Autodesk Inventor part; units mm, degrees
(part 8 of 15)
  arc A3405 (-52.178, -58.6781) -> (-52.178, -58.6019) centre (-52.178, -58.64) ccw
  arc A3406 (-55.022, -58.6019) -> (-55.022, -58.6781) centre (-55.022, -58.64) ccw
  line L1559 (-52.178, -58.64) -> (-52.178, -59.96)
  arc A3407 (-52.2161, -59.96) -> (-52.1399, -59.96) centre (-52.178, -59.96) ccw
  arc A3408 (-52.1399, -58.64) -> (-52.2161, -58.64) centre (-52.178, -58.64) ccw
  line L1560 (-52.178, -59.96) -> (-55.022, -59.96)
  arc A3409 (-55.022, -59.9219) -> (-55.022, -59.9981) centre (-55.022, -59.96) ccw
  arc A3410 (-52.178, -59.9981) -> (-52.178, -59.9219) centre (-52.178, -59.96) ccw
  line L1561 (-18.1, 57.4) -> (-18.1, 55)
  arc A3411 (-18.1317, 55) -> (-18.0682, 55) centre (-18.1, 55) ccw
  arc A3412 (-18.0682, 57.4) -> (-18.1317, 57.4) centre (-18.1, 57.4) ccw
  line L1562 (-18.1, 55) -> (-19.1, 55)
  arc A3413 (-19.1, 55.0318) -> (-19.1, 54.9683) centre (-19.1, 55) ccw
  arc A3414 (-18.1, 54.9683) -> (-18.1, 55.0318) centre (-18.1, 55) ccw
  line L1563 (-19.1, 55) -> (-19.1, 57.4)
  arc A3415 (-19.0682, 57.4) -> (-19.1317, 57.4) centre (-19.1, 57.4) ccw
  arc A3416 (-19.1317, 55) -> (-19.0682, 55) centre (-19.1, 55) ccw
  line L1564 (-19.1, 57.4) -> (-18.1, 57.4)
  arc A3417 (-18.1, 57.3683) -> (-18.1, 57.4317) centre (-18.1, 57.4) ccw
  arc A3418 (-19.1, 57.4317) -> (-19.1, 57.3683) centre (-19.1, 57.4) ccw
  line L1565 (-4.8, -82.3) -> (-4.8, -85.1)
  arc A3419 (-4.8318, -85.1) -> (-4.7682, -85.1) centre (-4.8, -85.1) ccw
  arc A3420 (-4.7682, -82.3) -> (-4.8318, -82.3) centre (-4.8, -82.3) ccw
  line L1566 (-6.6, -85.1) -> (-6.6, -82.3)
  arc A3421 (-6.5682, -82.3) -> (-6.6317, -82.3) centre (-6.6, -82.3) ccw
  arc A3422 (-6.6317, -85.1) -> (-6.5682, -85.1) centre (-6.6, -85.1) ccw
  line L1567 (-16.5, -87.6) -> (-16.5, -90.4)
  arc A3423 (-16.5318, -90.4) -> (-16.4683, -90.4) centre (-16.5001, -90.4) ccw
  arc A3424 (-16.4683, -87.6) -> (-16.5318, -87.6) centre (-16.5001, -87.6) ccw
  line L1568 (-18.3, -90.4) -> (-18.3, -87.6)
  arc A3425 (-18.2682, -87.6) -> (-18.3318, -87.6) centre (-18.3, -87.6) ccw
  arc A3426 (-18.3318, -90.4) -> (-18.2682, -90.4) centre (-18.3, -90.4) ccw
  line L1569 (-13.675, -20.475) -> (-13.675, -23.125)
  arc A3427 (-13.7004, -23.125) -> (-13.6496, -23.125) centre (-13.675, -23.125) ccw
  arc A3428 (-13.6496, -20.475) -> (-13.7004, -20.475) centre (-13.675, -20.475) ccw
  line L1570 (-12.125, -20.475) -> (-12.125, -23.125)
  arc A3429 (-12.1504, -23.125) -> (-12.0996, -23.125) centre (-12.125, -23.125) ccw
  arc A3430 (-12.0996, -20.475) -> (-12.1504, -20.475) centre (-12.125, -20.475) ccw
  line L1571 (-12.9, -21.3) -> (-12.4, -22.3)
  arc A3431 (-12.4454, -22.3227) -> (-12.3546, -22.2773) centre (-12.4, -22.3) ccw
  arc A3432 (-12.8546, -21.2773) -> (-12.9454, -21.3227) centre (-12.9, -21.3) ccw
  line L1572 (-12.4, -22.3) -> (-13.4, -22.3)
  arc A3433 (-13.4, -22.2492) -> (-13.4, -22.3508) centre (-13.4, -22.3) ccw
  arc A3434 (-12.4, -22.3508) -> (-12.4, -22.2492) centre (-12.4, -22.3) ccw
  line L1573 (-13.4, -22.3) -> (-12.9, -21.3)
  arc A3435 (-12.8546, -21.3227) -> (-12.9454, -21.2773) centre (-12.9, -21.3) ccw
  arc A3436 (-13.4454, -22.2773) -> (-13.3546, -22.3227) centre (-13.4, -22.3) ccw
  line L1574 (-12.4, -21.3) -> (-12.9, -21.3)
  arc A3437 (-12.9, -21.2492) -> (-12.9, -21.3508) centre (-12.9, -21.3) ccw
  arc A3438 (-12.4, -21.3508) -> (-12.4, -21.2492) centre (-12.4, -21.3) ccw
  line L1575 (-12.9, -21.3) -> (-13.4, -21.3)
  arc A3439 (-13.4, -21.2492) -> (-13.4, -21.3508) centre (-13.4, -21.3) ccw
  arc A3440 (-12.9, -21.3508) -> (-12.9, -21.2492) centre (-12.9, -21.3) ccw
  line L1576 (-15.6, 42.2) -> (-17.4, 42.2)
  arc A3441 (-17.4, 42.2317) -> (-17.4, 42.1683) centre (-17.4, 42.2) ccw
  arc A3442 (-15.6, 42.1683) -> (-15.6, 42.2317) centre (-15.6, 42.2) ccw
  line L1577 (-17.4, 43.6) -> (-15.6, 43.6)
  arc A3443 (-15.6, 43.5683) -> (-15.6, 43.6318) centre (-15.6, 43.6) ccw
  arc A3444 (-17.4, 43.6318) -> (-17.4, 43.5683) centre (-17.4, 43.6) ccw
  line L1578 (-17.4, 42.2) -> (-17.4, 43.6)
  arc A3445 (-17.3682, 43.6) -> (-17.4317, 43.6) centre (-17.4, 43.6) ccw
  arc A3446 (-17.4317, 42.2) -> (-17.3682, 42.2) centre (-17.4, 42.2) ccw
  line L1579 (-16.7, 42.23) -> (-16.7, 43.5)
  arc A3447 (-16.6682, 43.5) -> (-16.7317, 43.5) centre (-16.7, 43.5) ccw
  arc A3448 (-16.7317, 42.23) -> (-16.6682, 42.23) centre (-16.7, 42.23) ccw
  line L1580 (-15.6, 43.6) -> (-15.6, 42.2)
  arc A3449 (-15.6317, 42.2) -> (-15.5682, 42.2) centre (-15.6, 42.2) ccw
  arc A3450 (-15.5682, 43.6) -> (-15.6317, 43.6) centre (-15.6, 43.6) ccw
  line L1581 (16.64, -104.878) -> (17.96, -104.878)
  arc A3451 (17.96, -104.9161) -> (17.96, -104.8399) centre (17.96, -104.878) ccw
  arc A3452 (16.64, -104.8399) -> (16.64, -104.9161) centre (16.64, -104.878) ccw
  line L1582 (17.96, -104.878) -> (17.96, -107.722)
  arc A3453 (17.9219, -107.722) -> (17.9981, -107.722) centre (17.96, -107.722) ccw
  arc A3454 (17.9981, -104.878) -> (17.9219, -104.878) centre (17.96, -104.878) ccw
  line L1583 (17.96, -107.722) -> (16.64, -107.722)
  arc A3455 (16.64, -107.6839) -> (16.64, -107.7601) centre (16.64, -107.722) ccw
  arc A3456 (17.96, -107.7601) -> (17.96, -107.6839) centre (17.96, -107.722) ccw
  line L1584 (16.64, -107.722) -> (16.64, -104.878)
  arc A3457 (16.6781, -104.878) -> (16.6019, -104.878) centre (16.64, -104.878) ccw
  arc A3458 (16.6019, -107.722) -> (16.6781, -107.722) centre (16.64, -107.722) ccw
  line L1585 (66.55, 47.1) -> (69.05, 47.1)
  arc A3459 (69.05, 47.075) -> (69.05, 47.125) centre (69.05, 47.1) ccw
  arc A3460 (66.55, 47.125) -> (66.55, 47.075) centre (66.55, 47.1) ccw
  line L1586 (69.05, 46.1) -> (66.55, 46.1)
  arc A3461 (66.55, 46.125) -> (66.55, 46.075) centre (66.55, 46.1) ccw
  arc A3462 (69.05, 46.075) -> (69.05, 46.125) centre (69.05, 46.1) ccw
  line L1587 (69.05, 47.1) -> (69.05, 46.1)
  arc A3463 (69.025, 46.1) -> (69.075, 46.1) centre (69.05, 46.1) ccw
  arc A3464 (69.075, 47.1) -> (69.025, 47.1) centre (69.05, 47.1) ccw
  line L1588 (66.55, 46.1) -> (66.55, 47.1)
  arc A3465 (66.575, 47.1) -> (66.525, 47.1) centre (66.55, 47.1) ccw
  arc A3466 (66.525, 46.1) -> (66.575, 46.1) centre (66.55, 46.1) ccw
  arc A3467 (68.7, 46.75) -> (68.7, 46.85) centre (68.7, 46.8) ccw
  arc A3468 (68.7, 46.85) -> (68.7, 46.75) centre (68.7, 46.8) ccw
  line L1589 (64.6, 38.15) -> (64.6, 40.65)
  arc A3469 (64.625, 40.65) -> (64.575, 40.65) centre (64.6, 40.65) ccw
  arc A3470 (64.575, 38.15) -> (64.625, 38.15) centre (64.6, 38.15) ccw
  line L1590 (65.6, 40.65) -> (65.6, 38.15)
  arc A3471 (65.575, 38.15) -> (65.625, 38.15) centre (65.6, 38.15) ccw
  arc A3472 (65.625, 40.65) -> (65.575, 40.65) centre (65.6, 40.65) ccw
  line L1591 (64.6, 40.65) -> (65.6, 40.65)
  arc A3473 (65.6, 40.625) -> (65.6, 40.675) centre (65.6, 40.65) ccw
  arc A3474 (64.6, 40.675) -> (64.6, 40.625) centre (64.6, 40.65) ccw
  line L1592 (65.6, 38.15) -> (64.6, 38.15)
  arc A3475 (64.6, 38.175) -> (64.6, 38.125) centre (64.6, 38.15) ccw
  arc A3476 (65.6, 38.125) -> (65.6, 38.175) centre (65.6, 38.15) ccw
  arc A3477 (64.9, 40.25) -> (64.9, 40.35) centre (64.9, 40.3) ccw
  arc A3478 (64.9, 40.35) -> (64.9, 40.25) centre (64.9, 40.3) ccw
  line L1593 (-18.111, 52.3542) -> (-18.111, 50.0458)
  arc A3479 (-18.1427, 50.0458) -> (-18.0792, 50.0458) centre (-18.111, 50.0458) ccw
  arc A3480 (-18.0792, 52.3542) -> (-18.1427, 52.3542) centre (-18.111, 52.3542) ccw
  line L1594 (-18.111, 50.0458) -> (-19.089, 50.0458)
  arc A3481 (-19.089, 50.0775) -> (-19.089, 50.0141) centre (-19.089, 50.0458) ccw
  arc A3482 (-18.111, 50.0141) -> (-18.111, 50.0775) centre (-18.111, 50.0458) ccw
  line L1595 (-19.089, 50.0458) -> (-19.089, 52.3542)
  arc A3483 (-19.0572, 52.3542) -> (-19.1208, 52.3542) centre (-19.089, 52.3542) ccw
  arc A3484 (-19.1208, 50.0458) -> (-19.0572, 50.0458) centre (-19.089, 50.0458) ccw
  line L1596 (-19.089, 52.3542) -> (-18.111, 52.3542)
  arc A3485 (-18.111, 52.3225) -> (-18.111, 52.386) centre (-18.111, 52.3542) ccw
  arc A3486 (-19.089, 52.386) -> (-19.089, 52.3225) centre (-19.089, 52.3542) ccw
  line L1597 (-18.111, 54.6542) -> (-18.111, 52.3458)
  arc A3487 (-18.1427, 52.3458) -> (-18.0792, 52.3458) centre (-18.111, 52.3458) ccw
  arc A3488 (-18.0792, 54.6542) -> (-18.1427, 54.6542) centre (-18.111, 54.6542) ccw
  line L1598 (-18.111, 52.3458) -> (-19.089, 52.3458)
  arc A3489 (-19.089, 52.3776) -> (-19.089, 52.3141) centre (-19.089, 52.3458) ccw
  arc A3490 (-18.111, 52.3141) -> (-18.111, 52.3776) centre (-18.111, 52.3458) ccw
  line L1599 (-19.089, 52.3458) -> (-19.089, 54.6542)
  arc A3491 (-19.0572, 54.6542) -> (-19.1208, 54.6542) centre (-19.089, 54.6542) ccw
  arc A3492 (-19.1208, 52.3458) -> (-19.0572, 52.3458) centre (-19.089, 52.3458) ccw
  line L1600 (-19.089, 54.6542) -> (-18.111, 54.6542)
  arc A3493 (-18.111, 54.6225) -> (-18.111, 54.6859) centre (-18.111, 54.6542) ccw
  arc A3494 (-19.089, 54.6859) -> (-19.089, 54.6225) centre (-19.089, 54.6542) ccw
  line L1601 (-17.111, 56.0542) -> (-17.111, 53.7458)
  arc A3495 (-17.1427, 53.7458) -> (-17.0792, 53.7458) centre (-17.111, 53.7458) ccw
  arc A3496 (-17.0792, 56.0542) -> (-17.1427, 56.0542) centre (-17.111, 56.0542) ccw
  line L1602 (-17.111, 53.7458) -> (-18.089, 53.7458)
  arc A3497 (-18.089, 53.7775) -> (-18.089, 53.7141) centre (-18.089, 53.7458) ccw
  arc A3498 (-17.111, 53.7141) -> (-17.111, 53.7775) centre (-17.111, 53.7458) ccw
  line L1603 (-18.089, 53.7458) -> (-18.089, 56.0542)
  arc A3499 (-18.0572, 56.0542) -> (-18.1208, 56.0542) centre (-18.089, 56.0542) ccw
  arc A3500 (-18.1208, 53.7458) -> (-18.0572, 53.7458) centre (-18.089, 53.7458) ccw
  line L1604 (-18.089, 56.0542) -> (-17.111, 56.0542)
  arc A3501 (-17.111, 56.0225) -> (-17.111, 56.0859) centre (-17.111, 56.0542) ccw
  arc A3502 (-18.089, 56.0859) -> (-18.089, 56.0225) centre (-18.089, 56.0542) ccw
  line L1605 (-9.008, 3.184) -> (-9.008, 5.216)
  arc A3503 (-8.9572, 5.216) -> (-9.0588, 5.216) centre (-9.008, 5.216) ccw
  arc A3504 (-9.0588, 3.184) -> (-8.9572, 3.184) centre (-9.008, 3.184) ccw
  line L1606 (-9.008, 5.216) -> (-7.992, 5.216)
  arc A3505 (-7.992, 5.1652) -> (-7.992, 5.2668) centre (-7.992, 5.216) ccw
  arc A3506 (-9.008, 5.2668) -> (-9.008, 5.1652) centre (-9.008, 5.216) ccw
  line L1607 (-7.992, 5.216) -> (-7.992, 3.184)
  arc A3507 (-8.0428, 3.184) -> (-7.9412, 3.184) centre (-7.992, 3.184) ccw
  arc A3508 (-7.9412, 5.216) -> (-8.0428, 5.216) centre (-7.992, 5.216) ccw
  line L1608 (-7.992, 3.184) -> (-9.008, 3.184)
  arc A3509 (-9.008, 3.2348) -> (-9.008, 3.1332) centre (-9.008, 3.184) ccw
  arc A3510 (-7.992, 3.1332) -> (-7.992, 3.2348) centre (-7.992, 3.184) ccw
  line L1609 (-3.992, -3.784) -> (-3.992, -5.816)
  arc A3511 (-4.0428, -5.816) -> (-3.9412, -5.816) centre (-3.992, -5.816) ccw
  arc A3512 (-3.9412, -3.784) -> (-4.0428, -3.784) centre (-3.992, -3.784) ccw
  line L1610 (-3.992, -5.816) -> (-5.008, -5.816)
  arc A3513 (-5.008, -5.7652) -> (-5.008, -5.8668) centre (-5.008, -5.816) ccw
  arc A3514 (-3.992, -5.8668) -> (-3.992, -5.7652) centre (-3.992, -5.816) ccw
  line L1611 (-5.008, -5.816) -> (-5.008, -3.784)
  arc A3515 (-4.9572, -3.784) -> (-5.0588, -3.784) centre (-5.008, -3.784) ccw
  arc A3516 (-5.0588, -5.816) -> (-4.9572, -5.816) centre (-5.008, -5.816) ccw
  line L1612 (-5.008, -3.784) -> (-3.992, -3.784)
  arc A3517 (-3.992, -3.8348) -> (-3.992, -3.7332) centre (-3.992, -3.784) ccw
  arc A3518 (-5.008, -3.7332) -> (-5.008, -3.8348) centre (-5.008, -3.784) ccw
  line L1613 (-0.984, -4.808) -> (-3.016, -4.808)
  arc A3519 (-3.016, -4.7572) -> (-3.016, -4.8588) centre (-3.016, -4.808) ccw
  arc A3520 (-0.984, -4.8588) -> (-0.984, -4.7572) centre (-0.984, -4.808) ccw
  line L1614 (-3.016, -4.808) -> (-3.016, -3.792)
  arc A3521 (-2.9652, -3.792) -> (-3.0668, -3.792) centre (-3.016, -3.792) ccw
  arc A3522 (-3.0668, -4.808) -> (-2.9652, -4.808) centre (-3.016, -4.808) ccw
  line L1615 (-3.016, -3.792) -> (-0.984, -3.792)
  arc A3523 (-0.984, -3.8428) -> (-0.984, -3.7412) centre (-0.984, -3.792) ccw
  arc A3524 (-3.016, -3.7412) -> (-3.016, -3.8428) centre (-3.016, -3.792) ccw
  line L1616 (-0.984, -3.792) -> (-0.984, -4.808)
  arc A3525 (-1.0348, -4.808) -> (-0.9332, -4.808) centre (-0.984, -4.808) ccw
  arc A3526 (-0.9332, -3.792) -> (-1.0348, -3.792) centre (-0.984, -3.792) ccw
  line L1617 (-5.984, 5.192) -> (-8.016, 5.192)
  arc A3527 (-8.016, 5.2428) -> (-8.016, 5.1412) centre (-8.016, 5.192) ccw
  arc A3528 (-5.984, 5.1412) -> (-5.984, 5.2428) centre (-5.984, 5.192) ccw
  line L1618 (-8.016, 5.192) -> (-8.016, 6.208)
  arc A3529 (-7.9652, 6.208) -> (-8.0668, 6.208) centre (-8.016, 6.208) ccw
  arc A3530 (-8.0668, 5.192) -> (-7.9652, 5.192) centre (-8.016, 5.192) ccw
  line L1619 (-8.016, 6.208) -> (-5.984, 6.208)
  arc A3531 (-5.984, 6.1572) -> (-5.984, 6.2588) centre (-5.984, 6.208) ccw
  arc A3532 (-8.016, 6.2588) -> (-8.016, 6.1572) centre (-8.016, 6.208) ccw
  line L1620 (-5.984, 6.208) -> (-5.984, 5.192)
  arc A3533 (-6.0348, 5.192) -> (-5.9332, 5.192) centre (-5.984, 5.192) ccw
  arc A3534 (-5.9332, 6.208) -> (-6.0348, 6.208) centre (-5.984, 6.208) ccw
  line L1621 (-15.15, -102.15) -> (-15.15, -97.65)
  arc A3535 (-15.1182, -97.65) -> (-15.1817, -97.65) centre (-15.15, -97.65) ccw
  arc A3536 (-15.1817, -102.15) -> (-15.1182, -102.15) centre (-15.15, -102.15) ccw
  line L1622 (-15.15, -97.65) -> (-11.65, -97.65)
  arc A3537 (-11.65, -97.6817) -> (-11.65, -97.6182) centre (-11.65, -97.65) ccw
  arc A3538 (-15.15, -97.6182) -> (-15.15, -97.6817) centre (-15.15, -97.65) ccw
  line L1623 (-11.65, -102.15) -> (-15.15, -102.15)
  arc A3539 (-15.15, -102.1182) -> (-15.15, -102.1817) centre (-15.15, -102.15) ccw
  arc A3540 (-11.65, -102.1817) -> (-11.65, -102.1182) centre (-11.65, -102.15) ccw
  line L1624 (-11.65, -97.65) -> (-11.65, -102.15)
  arc A3541 (-11.6817, -102.15) -> (-11.6182, -102.15) centre (-11.65, -102.15) ccw
  arc A3542 (-11.6182, -97.65) -> (-11.6817, -97.65) centre (-11.65, -97.65) ccw
  arc A3543 (-14.7, -98.1) -> (-14.7, -97.9) centre (-14.7, -98) ccw
  arc A3544 (-14.7, -97.9) -> (-14.7, -98.1) centre (-14.7, -98) ccw
  line L1625 (19.6, -115) -> (16.6, -115)
  arc A3545 (16.6, -114.9682) -> (16.6, -115.0317) centre (16.6, -115) ccw
  arc A3546 (19.6, -115.0317) -> (19.6, -114.9682) centre (19.6, -115) ccw
  line L1626 (16.6, -112) -> (19.6, -112)
  arc A3547 (19.6, -112.0317) -> (19.6, -111.9682) centre (19.6, -112) ccw
  arc A3548 (16.6, -111.9682) -> (16.6, -112.0317) centre (16.6, -112) ccw
  line L1627 (19.6, -112) -> (19.6, -115)
  arc A3549 (19.5683, -115) -> (19.6318, -115) centre (19.6, -115) ccw
  arc A3550 (19.6318, -112) -> (19.5683, -112) centre (19.6, -112) ccw
  line L1628 (16.6, -115) -> (16.6, -112)
  arc A3551 (16.6318, -112) -> (16.5683, -112) centre (16.6, -112) ccw
  arc A3552 (16.5683, -115) -> (16.6318, -115) centre (16.6, -115) ccw
  arc A3553 (19.2, -112.5) -> (19.2, -112.3) centre (19.2, -112.4) ccw
  arc A3554 (19.2, -112.3) -> (19.2, -112.5) centre (19.2, -112.4) ccw
  line L1629 (-22.2, -23.7) -> (-22.2, -25.7)
  arc A3555 (-22.2318, -25.7) -> (-22.1682, -25.7) centre (-22.2, -25.7) ccw
  arc A3556 (-22.1682, -23.7) -> (-22.2318, -23.7) centre (-22.2, -23.7) ccw
  line L1630 (-24.2, -25.7) -> (-24.2, -23.7)
  arc A3557 (-24.1682, -23.7) -> (-24.2318, -23.7) centre (-24.2, -23.7) ccw
  arc A3558 (-24.2318, -25.7) -> (-24.1682, -25.7) centre (-24.2, -25.7) ccw
  arc A3559 (-21.9, -23.4) -> (-21.9, -23.2) centre (-21.9, -23.3) ccw
  arc A3560 (-21.9, -23.2) -> (-21.9, -23.4) centre (-21.9, -23.3) ccw
  line L1631 (-22.0888, 36.6332) -> (-22.0888, 38.7668)
  arc A3561 (-22.0507, 38.7668) -> (-22.1269, 38.7668) centre (-22.0888, 38.7668) ccw
  arc A3562 (-22.1269, 36.6332) -> (-22.0507, 36.6332) centre (-22.0888, 36.6332) ccw
  line L1632 (-22.0888, 38.7668) -> (-22.4952, 38.7668)
  arc A3563 (-22.4952, 38.8049) -> (-22.4952, 38.7287) centre (-22.4952, 38.7668) ccw
  arc A3564 (-22.0888, 38.7287) -> (-22.0888, 38.8049) centre (-22.0888, 38.7668) ccw
  line L1633 (-22.4952, 38.7668) -> (-22.5714, 38.7668)
  arc A3565 (-22.5714, 38.8049) -> (-22.5714, 38.7287) centre (-22.5714, 38.7668) ccw
  arc A3566 (-22.4952, 38.7287) -> (-22.4952, 38.8049) centre (-22.4952, 38.7668) ccw
  line L1634 (-22.5714, 38.7668) -> (-23.0286, 38.7668)
  arc A3567 (-23.0286, 38.8049) -> (-23.0286, 38.7287) centre (-23.0286, 38.7668) ccw
  arc A3568 (-22.5714, 38.7287) -> (-22.5714, 38.8049) centre (-22.5714, 38.7668) ccw
  line L1635 (-23.0286, 38.7668) -> (-23.1048, 38.7668)
  arc A3569 (-23.1048, 38.8049) -> (-23.1048, 38.7287) centre (-23.1048, 38.7668) ccw
  arc A3570 (-23.0286, 38.7287) -> (-23.0286, 38.8049) centre (-23.0286, 38.7668) ccw
  line L1636 (-23.1048, 38.7668) -> (-23.5112, 38.7668)
  arc A3571 (-23.5112, 38.8049) -> (-23.5112, 38.7287) centre (-23.5112, 38.7668) ccw
  arc A3572 (-23.1048, 38.7287) -> (-23.1048, 38.8049) centre (-23.1048, 38.7668) ccw
  arc A3573 (-23.1048, 38.7668) -> (-22.4952, 38.7668) centre (-22.8, 38.7668) ccw
  arc A3574 (-23.0667, 38.7668) -> (-23.1429, 38.7668) centre (-23.1048, 38.7668) ccw
  arc A3575 (-22.4571, 38.7668) -> (-22.5333, 38.7668) centre (-22.4952, 38.7668) ccw
  line L1637 (-23.0286, 36.6332) -> (-22.5714, 36.6332)
  arc A3576 (-22.5714, 36.5951) -> (-22.5714, 36.6713) centre (-22.5714, 36.6332) ccw
  arc A3577 (-23.0286, 36.6713) -> (-23.0286, 36.5951) centre (-23.0286, 36.6332) ccw
  line L1638 (-22.0888, 37.573) -> (-22.0888, 37.827)
  arc A3578 (-22.0507, 37.827) -> (-22.1269, 37.827) centre (-22.0888, 37.827) ccw
  arc A3579 (-22.1269, 37.573) -> (-22.0507, 37.573) centre (-22.0888, 37.573) ccw
  line L1639 (-22.5714, 38.7668) -> (-23.0286, 38.7668)
  arc A3580 (-23.0286, 38.8049) -> (-23.0286, 38.7287) centre (-23.0286, 38.7668) ccw
  arc A3581 (-22.5714, 38.7287) -> (-22.5714, 38.8049) centre (-22.5714, 38.7668) ccw
  line L1640 (-23.5112, 36.6332) -> (-22.0888, 36.6332)
  arc A3582 (-22.0888, 36.5951) -> (-22.0888, 36.6713) centre (-22.0888, 36.6332) ccw
  arc A3583 (-23.5112, 36.6713) -> (-23.5112, 36.5951) centre (-23.5112, 36.6332) ccw
  line L1641 (-23.5112, 38.7668) -> (-23.5112, 36.6332)
  arc A3584 (-23.5493, 36.6332) -> (-23.4731, 36.6332) centre (-23.5112, 36.6332) ccw
  arc A3585 (-23.4731, 38.7668) -> (-23.5493, 38.7668) centre (-23.5112, 38.7668) ccw
  line L1642 (-20.7, 46.9) -> (-20.7, 47.4)
  arc A3586 (-20.6682, 47.4) -> (-20.7317, 47.4) centre (-20.7, 47.4) ccw
  arc A3587 (-20.7317, 46.9) -> (-20.6682, 46.9) centre (-20.7, 46.9) ccw
  line L1643 (-20.7, 47.4) -> (-20.8, 47.4)
  arc A3588 (-20.8, 47.4317) -> (-20.8, 47.3683) centre (-20.8, 47.4) ccw
  arc A3589 (-20.7, 47.3683) -> (-20.7, 47.4317) centre (-20.7, 47.4) ccw
  line L1644 (-22.5, 46.9) -> (-22.5, 47.4)
  arc A3590 (-22.4682, 47.4) -> (-22.5317, 47.4) centre (-22.5, 47.4) ccw
  arc A3591 (-22.5317, 46.9) -> (-22.4682, 46.9) centre (-22.5, 46.9) ccw
  line L1645 (-22.5, 47.4) -> (-22.4, 47.4)
  arc A3592 (-22.4, 47.3683) -> (-22.4, 47.4317) centre (-22.4, 47.4) ccw
  arc A3593 (-22.5, 47.4317) -> (-22.5, 47.3683) centre (-22.5, 47.4) ccw
  line L1646 (-22.5, 45.3) -> (-22.5, 44.8)
  arc A3594 (-22.5317, 44.8) -> (-22.4682, 44.8) centre (-22.5, 44.8) ccw
  arc A3595 (-22.4682, 45.3) -> (-22.5317, 45.3) centre (-22.5, 45.3) ccw
  line L1647 (-22.5, 44.8) -> (-22.4, 44.8)
  arc A3596 (-22.4, 44.7683) -> (-22.4, 44.8317) centre (-22.4, 44.8) ccw
  arc A3597 (-22.5, 44.8317) -> (-22.5, 44.7683) centre (-22.5, 44.8) ccw
  line L1648 (-20.7, 45.3) -> (-20.7, 44.8)
  arc A3598 (-20.7317, 44.8) -> (-20.6682, 44.8) centre (-20.7, 44.8) ccw
  arc A3599 (-20.6682, 45.3) -> (-20.7317, 45.3) centre (-20.7, 45.3) ccw
  line L1649 (-20.7, 44.8) -> (-20.8, 44.8)
  arc A3600 (-20.8, 44.8317) -> (-20.8, 44.7683) centre (-20.8, 44.8) ccw
  arc A3601 (-20.7, 44.7683) -> (-20.7, 44.8317) centre (-20.7, 44.8) ccw
  arc A3602 (-20.2, 45.4293) -> (-20.2, 45.5707) centre (-20.2, 45.5) ccw
  arc A3603 (-20.2, 45.5707) -> (-20.2, 45.4293) centre (-20.2, 45.5) ccw
  line L1650 (-24.25, 43.05) -> (-23.51, 43.05)
  arc A3604 (-23.51, 43.0183) -> (-23.51, 43.0817) centre (-23.51, 43.05) ccw
  arc A3605 (-24.25, 43.0817) -> (-24.25, 43.0183) centre (-24.25, 43.05) ccw
  line L1651 (-23.51, 43.05) -> (-23.35, 42.89)
  arc A3606 (-23.3725, 42.8675) -> (-23.3275, 42.9125) centre (-23.35, 42.89) ccw
  arc A3607 (-23.4875, 43.0725) -> (-23.5325, 43.0275) centre (-23.51, 43.05) ccw
  line L1652 (-23.35, 42.89) -> (-23.35, 42.15)
  arc A3608 (-23.3817, 42.15) -> (-23.3182, 42.15) centre (-23.35, 42.15) ccw
  arc A3609 (-23.3182, 42.89) -> (-23.3817, 42.89) centre (-23.35, 42.89) ccw
  line L1653 (-23.35, 42.15) -> (-24.25, 42.15)
  arc A3610 (-24.25, 42.1817) -> (-24.25, 42.1183) centre (-24.25, 42.15) ccw
  arc A3611 (-23.35, 42.1183) -> (-23.35, 42.1817) centre (-23.35, 42.15) ccw
  line L1654 (-24.25, 42.15) -> (-24.25, 43.05)
  arc A3612 (-24.2182, 43.05) -> (-24.2817, 43.05) centre (-24.25, 43.05) ccw
  arc A3613 (-24.2817, 42.15) -> (-24.2182, 42.15) centre (-24.25, 42.15) ccw
  line L1655 (-20.15, 42.85) -> (-19.41, 42.85)
  arc A3614 (-19.41, 42.8183) -> (-19.41, 42.8818) centre (-19.41, 42.85) ccw
  arc A3615 (-20.15, 42.8818) -> (-20.15, 42.8183) centre (-20.15, 42.85) ccw
  line L1656 (-19.41, 42.85) -> (-19.25, 42.69)
  arc A3616 (-19.2725, 42.6675) -> (-19.2275, 42.7125) centre (-19.25, 42.69) ccw
  arc A3617 (-19.3875, 42.8725) -> (-19.4325, 42.8275) centre (-19.41, 42.85) ccw
  line L1657 (-19.25, 42.69) -> (-19.25, 41.95)
  arc A3618 (-19.2818, 41.95) -> (-19.2183, 41.95) centre (-19.2501, 41.95) ccw
  arc A3619 (-19.2183, 42.69) -> (-19.2818, 42.69) centre (-19.2501, 42.69) ccw
  line L1658 (-19.25, 41.95) -> (-20.15, 41.95)
  arc A3620 (-20.15, 41.9817) -> (-20.15, 41.9183) centre (-20.15, 41.95) ccw
  arc A3621 (-19.25, 41.9183) -> (-19.25, 41.9817) centre (-19.25, 41.95) ccw
  line L1659 (-20.15, 41.95) -> (-20.15, 42.85)
  arc A3622 (-20.1182, 42.85) -> (-20.1817, 42.85) centre (-20.15, 42.85) ccw
  arc A3623 (-20.1817, 41.95) -> (-20.1182, 41.95) centre (-20.15, 41.95) ccw
  line L1660 (4.8, -41.3) -> (1.8, -41.3)
  arc A3624 (1.8, -41.2683) -> (1.8, -41.3318) centre (1.8, -41.3001) ccw
  arc A3625 (4.8, -41.3318) -> (4.8, -41.2683) centre (4.8, -41.3001) ccw
  line L1661 (1.8, -38.3) -> (4.8, -38.3)
  arc A3626 (4.8, -38.3317) -> (4.8, -38.2682) centre (4.8, -38.3) ccw
  arc A3627 (1.8, -38.2682) -> (1.8, -38.3317) centre (1.8, -38.3) ccw
  line L1662 (4.8, -38.3) -> (4.8, -41.3)
  arc A3628 (4.7683, -41.3) -> (4.8318, -41.3) centre (4.8, -41.3) ccw
  arc A3629 (4.8318, -38.3) -> (4.7683, -38.3) centre (4.8, -38.3) ccw
  line L1663 (1.8, -41.3) -> (1.8, -38.3)
  arc A3630 (1.8318, -38.3) -> (1.7683, -38.3) centre (1.8, -38.3) ccw
  arc A3631 (1.7683, -41.3) -> (1.8318, -41.3) centre (1.8, -41.3) ccw
  arc A3632 (4.4, -38.8414) -> (4.4, -38.5586) centre (4.4, -38.7) ccw
  arc A3633 (4.4, -38.5586) -> (4.4, -38.8414) centre (4.4, -38.7) ccw
  line L1664 (8.7, -41.3) -> (5.7, -41.3)
  arc A3634 (5.7, -41.2683) -> (5.7, -41.3318) centre (5.7, -41.3001) ccw
  arc A3635 (8.7, -41.3318) -> (8.7, -41.2683) centre (8.7, -41.3001) ccw
  line L1665 (5.7, -38.3) -> (8.7, -38.3)
  arc A3636 (8.7, -38.3317) -> (8.7, -38.2682) centre (8.7, -38.3) ccw
  arc A3637 (5.7, -38.2682) -> (5.7, -38.3317) centre (5.7, -38.3) ccw
  line L1666 (8.7, -38.3) -> (8.7, -41.3)
  arc A3638 (8.6682, -41.3) -> (8.7318, -41.3) centre (8.7, -41.3) ccw
  arc A3639 (8.7318, -38.3) -> (8.6682, -38.3) centre (8.7, -38.3) ccw
  line L1667 (5.7, -41.3) -> (5.7, -38.3)
  arc A3640 (5.7318, -38.3) -> (5.6682, -38.3) centre (5.7, -38.3) ccw
  arc A3641 (5.6682, -41.3) -> (5.7318, -41.3) centre (5.7, -41.3) ccw
  arc A3642 (8.3, -38.8414) -> (8.3, -38.5586) centre (8.3, -38.7) ccw
  arc A3643 (8.3, -38.5586) -> (8.3, -38.8414) centre (8.3, -38.7) ccw
  line L1668 (24.3336, -36.4042) -> (20.0664, -36.4042)
  arc A3644 (20.0664, -36.3661) -> (20.0664, -36.4423) centre (20.0664, -36.4042) ccw
  arc A3645 (24.3336, -36.4423) -> (24.3336, -36.3661) centre (24.3336, -36.4042) ccw
  line L1669 (20.0664, -45.3958) -> (24.3336, -45.3958)
  arc A3646 (24.3336, -45.4339) -> (24.3336, -45.3577) centre (24.3336, -45.3958) ccw
  arc A3647 (20.0664, -45.3577) -> (20.0664, -45.4339) centre (20.0664, -45.3958) ccw
  arc A3648 (25.01, -46.04) -> (25.01, -45.64) centre (25.01, -45.84) ccw
  arc A3649 (25.01, -45.64) -> (25.01, -46.04) centre (25.01, -45.84) ccw
  line L1670 (13, -48.3) -> (18, -48.3)
  arc A3650 (18, -48.3381) -> (18, -48.2619) centre (18, -48.3) ccw
  arc A3651 (13, -48.2619) -> (13, -48.3381) centre (13, -48.3) ccw
  line L1671 (18, -43.9) -> (18, -48.3)
  arc A3652 (17.9619, -48.3) -> (18.0381, -48.3) centre (18, -48.3) ccw
  arc A3653 (18.0381, -43.9) -> (17.9619, -43.9) centre (18, -43.9) ccw
  line L1672 (18, -43.9) -> (13, -43.9)
  arc A3654 (13, -43.8619) -> (13, -43.9381) centre (13, -43.9) ccw
  arc A3655 (18, -43.9381) -> (18, -43.8619) centre (18, -43.9) ccw
  line L1673 (13, -48.3) -> (13, -43.9)
  arc A3656 (13.0381, -43.9) -> (12.9619, -43.9) centre (13, -43.9) ccw
  arc A3657 (12.9619, -48.3) -> (13.0381, -48.3) centre (13, -48.3) ccw
  line L1674 (13.214, -48.1542) -> (17.786, -48.1542)
  arc A3658 (17.786, -48.1669) -> (17.786, -48.1415) centre (17.786, -48.1542) ccw
  arc A3659 (13.214, -48.1415) -> (13.214, -48.1669) centre (13.214, -48.1542) ccw
  line L1675 (17.786, -44.0458) -> (17.786, -48.1542)
  arc A3660 (17.7733, -48.1542) -> (17.7987, -48.1542) centre (17.786, -48.1542) ccw
  arc A3661 (17.7987, -44.0458) -> (17.7733, -44.0458) centre (17.786, -44.0458) ccw
  line L1676 (17.786, -44.0458) -> (13.214, -44.0458)
  arc A3662 (13.214, -44.0331) -> (13.214, -44.0585) centre (13.214, -44.0458) ccw
  arc A3663 (17.786, -44.0585) -> (17.786, -44.0331) centre (17.786, -44.0458) ccw
  line L1677 (13.214, -48.1542) -> (13.214, -44.0458)
  arc A3664 (13.2267, -44.0458) -> (13.2013, -44.0458) centre (13.214, -44.0458) ccw
  arc A3665 (13.2013, -48.1542) -> (13.2267, -48.1542) centre (13.214, -48.1542) ccw
  arc A3666 (13.8744, -47.7764) -> (13.8744, -46.862) centre (13.8744, -47.3192) ccw
  arc A3667 (13.8744, -46.862) -> (13.8744, -47.7764) centre (13.8744, -47.3192) ccw
  line L1678 (63.35, 54.615) -> (63.35, 54.95)
  arc A3668 (63.375, 54.95) -> (63.325, 54.95) centre (63.35, 54.95) ccw
  arc A3669 (63.325, 54.615) -> (63.375, 54.615) centre (63.35, 54.615) ccw
  line L1679 (63.35, 54.95) -> (64.35, 54.95)
  arc A3670 (64.35, 54.925) -> (64.35, 54.975) centre (64.35, 54.95) ccw
  arc A3671 (63.35, 54.975) -> (63.35, 54.925) centre (63.35, 54.95) ccw
  line L1680 (63.35, 50.7) -> (63.35, 50.45)
  arc A3672 (63.325, 50.45) -> (63.375, 50.45) centre (63.35, 50.45) ccw
  arc A3673 (63.375, 50.7) -> (63.325, 50.7) centre (63.35, 50.7) ccw
  line L1681 (63.35, 50.45) -> (64.35, 50.45)
  arc A3674 (64.35, 50.425) -> (64.35, 50.475) centre (64.35, 50.45) ccw
  arc A3675 (63.35, 50.475) -> (63.35, 50.425) centre (63.35, 50.45) ccw
  line L1682 (65.35, 54.95) -> (66.35, 54.95)
  arc A3676 (66.35, 54.925) -> (66.35, 54.975) centre (66.35, 54.95) ccw
  arc A3677 (65.35, 54.975) -> (65.35, 54.925) centre (65.35, 54.95) ccw
  line L1683 (66.35, 54.95) -> (66.35, 54.615)
  arc A3678 (66.325, 54.615) -> (66.375, 54.615) centre (66.35, 54.615) ccw
  arc A3679 (66.375, 54.95) -> (66.325, 54.95) centre (66.35, 54.95) ccw
  line L1684 (66.35, 50.785) -> (66.35, 50.45)
  arc A3680 (66.325, 50.45) -> (66.375, 50.45) centre (66.35, 50.45) ccw
  arc A3681 (66.375, 50.785) -> (66.325, 50.785) centre (66.35, 50.785) ccw
  line L1685 (66.35, 50.45) -> (65.35, 50.45)
  arc A3682 (65.35, 50.475) -> (65.35, 50.425) centre (65.35, 50.45) ccw
  arc A3683 (66.35, 50.425) -> (66.35, 50.475) centre (66.35, 50.45) ccw
  arc A3684 (66.65, 54.8) -> (66.55, 54.8) centre (66.6, 54.8) ccw
  arc A3685 (66.625, 54.8) -> (66.675, 54.8) centre (66.65, 54.8) ccw
  arc A3686 (66.525, 54.8) -> (66.575, 54.8) centre (66.55, 54.8) ccw
  arc A3687 (66.55, 54.8) -> (66.65, 54.8) centre (66.6, 54.8) ccw
  arc A3688 (66.575, 54.8) -> (66.525, 54.8) centre (66.55, 54.8) ccw
  arc A3689 (66.675, 54.8) -> (66.625, 54.8) centre (66.65, 54.8) ccw
  line L1686 (0.7838, 56.1162) -> (0.7838, 55.7098)
  arc A3690 (0.7457, 55.7098) -> (0.8219, 55.7098) centre (0.7838, 55.7098) ccw
  arc A3691 (0.8219, 56.1162) -> (0.7457, 56.1162) centre (0.7838, 56.1162) ccw
  line L1687 (0.7838, 50.8838) -> (1.1902, 50.8838)
  arc A3692 (1.1902, 50.8457) -> (1.1902, 50.9219) centre (1.1902, 50.8838) ccw
  arc A3693 (0.7838, 50.9219) -> (0.7838, 50.8457) centre (0.7838, 50.8838) ccw
  line L1688 (6.0162, 50.8838) -> (6.0162, 51.2902)
  arc A3694 (6.0543, 51.2902) -> (5.9781, 51.2902) centre (6.0162, 51.2902) ccw
  arc A3695 (5.9781, 50.8838) -> (6.0543, 50.8838) centre (6.0162, 50.8838) ccw
  line L1689 (6.0162, 56.1162) -> (5.6098, 56.1162)
  arc A3696 (5.6098, 56.1543) -> (5.6098, 56.0781) centre (5.6098, 56.1162) ccw
  arc A3697 (6.0162, 56.0781) -> (6.0162, 56.1543) centre (6.0162, 56.1162) ccw
  line L1690 (1.1902, 56.1162) -> (0.7838, 56.1162)
  arc A3698 (0.7838, 56.1543) -> (0.7838, 56.0781) centre (0.7838, 56.1162) ccw
  arc A3699 (1.1902, 56.0781) -> (1.1902, 56.1543) centre (1.1902, 56.1162) ccw
  line L1691 (0.7838, 51.2902) -> (0.7838, 50.8838)
  arc A3700 (0.7457, 50.8838) -> (0.8219, 50.8838) centre (0.7838, 50.8838) ccw
  arc A3701 (0.8219, 51.2902) -> (0.7457, 51.2902) centre (0.7838, 51.2902) ccw
  line L1692 (5.6098, 50.8838) -> (6.0162, 50.8838)
  arc A3702 (6.0162, 50.8457) -> (6.0162, 50.9219) centre (6.0162, 50.8838) ccw
  arc A3703 (5.6098, 50.9219) -> (5.6098, 50.8457) centre (5.6098, 50.8838) ccw
  line L1693 (6.0162, 55.7098) -> (6.0162, 56.1162)
  arc A3704 (6.0543, 56.1162) -> (5.9781, 56.1162) centre (6.0162, 56.1162) ccw
  arc A3705 (5.9781, 55.7098) -> (6.0543, 55.7098) centre (6.0162, 55.7098) ccw
  arc A3706 (5.5, 55.4882) -> (5.5, 55.7118) centre (5.5, 55.6) ccw
  arc A3707 (5.5, 55.7118) -> (5.5, 55.4882) centre (5.5, 55.6) ccw
  line L1694 (3.3504, 38.0662) -> (2.7662, 38.0662)
  arc A3708 (2.7662, 38.117) -> (2.7662, 38.0154) centre (2.7662, 38.0662) ccw
  arc A3709 (3.3504, 38.0154) -> (3.3504, 38.117) centre (3.3504, 38.0662) ccw
  line L1695 (2.7662, 38.0662) -> (2.7662, 38.6504)
  arc A3710 (2.817, 38.6504) -> (2.7154, 38.6504) centre (2.7662, 38.6504) ccw
  arc A3711 (2.7154, 38.0662) -> (2.817, 38.0662) centre (2.7662, 38.0662) ccw
  line L1696 (2.7662, 45.229) -> (2.7662, 45.5338)
  arc A3712 (2.817, 45.5338) -> (2.7154, 45.5338) centre (2.7662, 45.5338) ccw
  arc A3713 (2.7154, 45.229) -> (2.817, 45.229) centre (2.7662, 45.229) ccw
  line L1697 (3.071, 45.5338) -> (2.7662, 45.5338)
  arc A3714 (2.7662, 45.5846) -> (2.7662, 45.483) centre (2.7662, 45.5338) ccw
  arc A3715 (3.071, 45.483) -> (3.071, 45.5846) centre (3.071, 45.5338) ccw
  line L1698 (10.2338, 45.5338) -> (9.929, 45.5338)
  arc A3716 (9.929, 45.5846) -> (9.929, 45.483) centre (9.929, 45.5338) ccw
  arc A3717 (10.2338, 45.483) -> (10.2338, 45.5846) centre (10.2338, 45.5338) ccw
  line L1699 (10.2338, 45.229) -> (10.2338, 45.5338)
  arc A3718 (10.2846, 45.5338) -> (10.183, 45.5338) centre (10.2338, 45.5338) ccw
  arc A3719 (10.183, 45.229) -> (10.2846, 45.229) centre (10.2338, 45.229) ccw
  line L1700 (10.2338, 38.0662) -> (9.929, 38.0662)
  arc A3720 (9.929, 38.117) -> (9.929, 38.0154) centre (9.929, 38.0662) ccw
  arc A3721 (10.2338, 38.0154) -> (10.2338, 38.117) centre (10.2338, 38.0662) ccw
  line L1701 (10.2338, 38.0662) -> (10.2338, 38.371)
  arc A3722 (10.2846, 38.371) -> (10.183, 38.371) centre (10.2338, 38.371) ccw
  arc A3723 (10.183, 38.0662) -> (10.2846, 38.0662) centre (10.2338, 38.0662) ccw
  arc A3724 (3.833, 39.4124) -> (3.833, 38.8282) centre (3.833, 39.1203) ccw
  arc A3725 (3.833, 39.387) -> (3.833, 39.4378) centre (3.833, 39.4124) ccw
  arc A3726 (3.833, 38.8028) -> (3.833, 38.8536) centre (3.833, 38.8282) ccw
  arc A3727 (3.833, 38.8282) -> (3.833, 39.4124) centre (3.833, 39.1203) ccw
  arc A3728 (3.833, 38.8536) -> (3.833, 38.8028) centre (3.833, 38.8282) ccw
  arc A3729 (3.833, 39.4378) -> (3.833, 39.387) centre (3.833, 39.4124) ccw
  line L1702 (19, -53.8) -> (19, -58.8)
  arc A3730 (18.9619, -58.8) -> (19.0381, -58.8) centre (19, -58.8) ccw
  arc A3731 (19.0381, -53.8) -> (18.9619, -53.8) centre (19, -53.8) ccw
  line L1703 (23.4, -58.8) -> (19, -58.8)
  arc A3732 (19, -58.7619) -> (19, -58.8381) centre (19, -58.8) ccw
  arc A3733 (23.4, -58.8381) -> (23.4, -58.7619) centre (23.4, -58.8) ccw
  line L1704 (23.4, -58.8) -> (23.4, -53.8)
  arc A3734 (23.4381, -53.8) -> (23.3619, -53.8) centre (23.4, -53.8) ccw
  arc A3735 (23.3619, -58.8) -> (23.4381, -58.8) centre (23.4, -58.8) ccw
  line L1705 (19, -53.8) -> (23.4, -53.8)
  arc A3736 (23.4, -53.8381) -> (23.4, -53.7619) centre (23.4, -53.8) ccw
  arc A3737 (19, -53.7619) -> (19, -53.8381) centre (19, -53.8) ccw
  line L1706 (19.1458, -54.014) -> (19.1458, -58.586)
  arc A3738 (19.1331, -58.586) -> (19.1585, -58.586) centre (19.1458, -58.586) ccw
  arc A3739 (19.1585, -54.014) -> (19.1331, -54.014) centre (19.1458, -54.014) ccw
  line L1707 (23.2542, -58.586) -> (19.1458, -58.586)
  arc A3740 (19.1458, -58.5733) -> (19.1458, -58.5987) centre (19.1458, -58.586) ccw
  arc A3741 (23.2542, -58.5987) -> (23.2542, -58.5733) centre (23.2542, -58.586) ccw
  line L1708 (23.2542, -58.586) -> (23.2542, -54.014)
  arc A3742 (23.2669, -54.014) -> (23.2415, -54.014) centre (23.2542, -54.014) ccw
  arc A3743 (23.2415, -58.586) -> (23.2669, -58.586) centre (23.2542, -58.586) ccw
  line L1709 (19.1458, -54.014) -> (23.2542, -54.014)
  arc A3744 (23.2542, -54.0267) -> (23.2542, -54.0013) centre (23.2542, -54.014) ccw
  arc A3745 (19.1458, -54.0013) -> (19.1458, -54.0267) centre (19.1458, -54.014) ccw
  arc A3746 (19.9808, -55.1316) -> (19.9808, -54.2172) centre (19.9808, -54.6744) ccw
  arc A3747 (19.9808, -54.2172) -> (19.9808, -55.1316) centre (19.9808, -54.6744) ccw
  line L1710 (-13.5, 50.75) -> (-16.7, 50.75)
  arc A3748 (-16.7, 50.7818) -> (-16.7, 50.7183) centre (-16.7, 50.75) ccw
  arc A3749 (-13.5, 50.7183) -> (-13.5, 50.7818) centre (-13.5, 50.75) ccw
  line L1711 (-16.7, 50.75) -> (-16.7, 53.25)
  arc A3750 (-16.6682, 53.25) -> (-16.7317, 53.25) centre (-16.7, 53.25) ccw
  arc A3751 (-16.7317, 50.75) -> (-16.6682, 50.75) centre (-16.7, 50.75) ccw
  line L1712 (-13.5, 53.25) -> (-13.5, 50.75)
  arc A3752 (-13.5318, 50.75) -> (-13.4683, 50.75) centre (-13.5001, 50.75) ccw
  arc A3753 (-13.4683, 53.25) -> (-13.5318, 53.25) centre (-13.5001, 53.25) ccw
  line L1713 (-16.7, 53.25) -> (-13.5, 53.25)
  arc A3754 (-13.5, 53.2183) -> (-13.5, 53.2818) centre (-13.5, 53.25) ccw
  arc A3755 (-16.7, 53.2818) -> (-16.7, 53.2183) centre (-16.7, 53.25) ccw
  line L1714 (-12.875, -36.61) -> (-7.925, -36.61)
  arc A3756 (-7.925, -36.6417) -> (-7.925, -36.5782) centre (-7.925, -36.61) ccw
  arc A3757 (-12.875, -36.5782) -> (-12.875, -36.6417) centre (-12.875, -36.61) ccw
  line L1715 (-7.925, -39.79) -> (-12.875, -39.79)
  arc A3758 (-12.875, -39.7582) -> (-12.875, -39.8218) centre (-12.875, -39.79) ccw
  arc A3759 (-7.925, -39.8218) -> (-7.925, -39.7582) centre (-7.925, -39.79) ccw
  line L1716 (-12.875, -39.79) -> (-12.875, -36.61)
  arc A3760 (-12.8433, -36.61) -> (-12.9068, -36.61) centre (-12.8751, -36.61) ccw
  arc A3761 (-12.9068, -39.79) -> (-12.8433, -39.79) centre (-12.8751, -39.79) ccw
  line L1717 (-7.925, -36.61) -> (-7.925, -39.79)
  arc A3762 (-7.9568, -39.79) -> (-7.8932, -39.79) centre (-7.925, -39.79) ccw
  arc A3763 (-7.8932, -36.61) -> (-7.9568, -36.61) centre (-7.925, -36.61) ccw
  arc A3764 (-11.4, -39.165) -> (-11.4, -38.965) centre (-11.4, -39.065) ccw
  arc A3765 (-11.4, -38.965) -> (-11.4, -39.165) centre (-11.4, -39.065) ccw
  arc A3766 (-11.4, -37.435) -> (-11.4, -37.235) centre (-11.4, -37.335) ccw
  arc A3767 (-11.4, -37.235) -> (-11.4, -37.435) centre (-11.4, -37.335) ccw
  line L1718 (-3.375, -36.61) -> (1.575, -36.61)
  arc A3768 (1.575, -36.6417) -> (1.575, -36.5782) centre (1.575, -36.61) ccw
  arc A3769 (-3.375, -36.5782) -> (-3.375, -36.6417) centre (-3.375, -36.61) ccw
  line L1719 (1.575, -39.79) -> (-3.375, -39.79)
  arc A3770 (-3.375, -39.7582) -> (-3.375, -39.8218) centre (-3.375, -39.79) ccw
  arc A3771 (1.575, -39.8218) -> (1.575, -39.7582) centre (1.575, -39.79) ccw
  line L1720 (-3.375, -39.79) -> (-3.375, -36.61)
  arc A3772 (-3.3433, -36.61) -> (-3.4068, -36.61) centre (-3.3751, -36.61) ccw
  arc A3773 (-3.4068, -39.79) -> (-3.3433, -39.79) centre (-3.3751, -39.79) ccw
  line L1721 (1.575, -36.61) -> (1.575, -39.79)
  arc A3774 (1.5432, -39.79) -> (1.6068, -39.79) centre (1.575, -39.79) ccw
  arc A3775 (1.6068, -36.61) -> (1.5432, -36.61) centre (1.575, -36.61) ccw
  arc A3776 (-1.9, -39.165) -> (-1.9, -38.965) centre (-1.9, -39.065) ccw
  arc A3777 (-1.9, -38.965) -> (-1.9, -39.165) centre (-1.9, -39.065) ccw
  arc A3778 (-1.9, -37.435) -> (-1.9, -37.235) centre (-1.9, -37.335) ccw
  arc A3779 (-1.9, -37.235) -> (-1.9, -37.435) centre (-1.9, -37.335) ccw
  line L1722 (-19.1, -80.71) -> (-18.9, -80.71)
  arc A3780 (-18.9, -80.76) -> (-18.9, -80.66) centre (-18.9, -80.71) ccw
  arc A3781 (-19.1, -80.66) -> (-19.1, -80.76) centre (-19.1, -80.71) ccw
  line L1723 (-18.9, -80.71) -> (-18.9, -75.51)
  arc A3782 (-18.85, -75.51) -> (-18.95, -75.51) centre (-18.9, -75.51) ccw
  arc A3783 (-18.95, -80.71) -> (-18.85, -80.71) centre (-18.9, -80.71) ccw
  line L1724 (-18.9, -75.51) -> (-19.1, -75.51)
  arc A3784 (-19.1, -75.46) -> (-19.1, -75.56) centre (-19.1, -75.51) ccw
  arc A3785 (-18.9, -75.56) -> (-18.9, -75.46) centre (-18.9, -75.51) ccw
  line L1725 (-25.9, -75.51) -> (-26.1, -75.51)
  arc A3786 (-26.1, -75.46) -> (-26.1, -75.56) centre (-26.1, -75.51) ccw
  arc A3787 (-25.9, -75.56) -> (-25.9, -75.46) centre (-25.9, -75.51) ccw
  line L1726 (-26.1, -75.51) -> (-26.1, -80.71)
  arc A3788 (-26.15, -80.71) -> (-26.05, -80.71) centre (-26.1, -80.71) ccw
  arc A3789 (-26.05, -75.51) -> (-26.15, -75.51) centre (-26.1, -75.51) ccw
  line L1727 (-26.1, -80.71) -> (-25.9, -80.71)
  arc A3790 (-25.9, -80.76) -> (-25.9, -80.66) centre (-25.9, -80.71) ccw
  arc A3791 (-26.1, -80.66) -> (-26.1, -80.76) centre (-26.1, -80.71) ccw
  line L1728 (-25.9, -13.89) -> (-26.1, -13.89)
  arc A3792 (-26.1, -13.84) -> (-26.1, -13.94) centre (-26.1, -13.89) ccw
  arc A3793 (-25.9, -13.94) -> (-25.9, -13.84) centre (-25.9, -13.89) ccw
  line L1729 (-26.1, -13.89) -> (-26.1, -19.09)
  arc A3794 (-26.15, -19.09) -> (-26.05, -19.09) centre (-26.1, -19.09) ccw
  arc A3795 (-26.05, -13.89) -> (-26.15, -13.89) centre (-26.1, -13.89) ccw
  line L1730 (-26.1, -19.09) -> (-25.9, -19.09)
  arc A3796 (-25.9, -19.14) -> (-25.9, -19.04) centre (-25.9, -19.09) ccw
  arc A3797 (-26.1, -19.04) -> (-26.1, -19.14) centre (-26.1, -19.09) ccw
  line L1731 (-19.1, -19.09) -> (-18.9, -19.09)
  arc A3798 (-18.9, -19.14) -> (-18.9, -19.04) centre (-18.9, -19.09) ccw
  arc A3799 (-19.1, -19.04) -> (-19.1, -19.14) centre (-19.1, -19.09) ccw
  line L1732 (-18.9, -19.09) -> (-18.9, -13.89)
  arc A3800 (-18.85, -13.89) -> (-18.95, -13.89) centre (-18.9, -13.89) ccw
  arc A3801 (-18.95, -19.09) -> (-18.85, -19.09) centre (-18.9, -19.09) ccw
  line L1733 (-18.9, -13.89) -> (-19.1, -13.89)
  arc A3802 (-19.1, -13.84) -> (-19.1, -13.94) centre (-19.1, -13.89) ccw
  arc A3803 (-18.9, -13.94) -> (-18.9, -13.84) centre (-18.9, -13.89) ccw
  line L1734 (-25.9, 16.71) -> (-26.1, 16.71)
  arc A3804 (-26.1, 16.76) -> (-26.1, 16.66) centre (-26.1, 16.71) ccw
  arc A3805 (-25.9, 16.66) -> (-25.9, 16.76) centre (-25.9, 16.71) ccw
  line L1735 (-26.1, 16.71) -> (-26.1, 11.51)
  arc A3806 (-26.15, 11.51) -> (-26.05, 11.51) centre (-26.1, 11.51) ccw
  arc A3807 (-26.05, 16.71) -> (-26.15, 16.71) centre (-26.1, 16.71) ccw
  line L1736 (-26.1, 11.51) -> (-25.9, 11.51)
  arc A3808 (-25.9, 11.46) -> (-25.9, 11.56) centre (-25.9, 11.51) ccw
  arc A3809 (-26.1, 11.56) -> (-26.1, 11.46) centre (-26.1, 11.51) ccw
  line L1737 (-19.1, 11.51) -> (-18.9, 11.51)
  arc A3810 (-18.9, 11.46) -> (-18.9, 11.56) centre (-18.9, 11.51) ccw
  arc A3811 (-19.1, 11.56) -> (-19.1, 11.46) centre (-19.1, 11.51) ccw
  line L1738 (-18.9, 11.51) -> (-18.9, 16.71)
  arc A3812 (-18.85, 16.71) -> (-18.95, 16.71) centre (-18.9, 16.71) ccw
  arc A3813 (-18.95, 11.51) -> (-18.85, 11.51) centre (-18.9, 11.51) ccw
  line L1739 (-18.9, 16.71) -> (-19.1, 16.71)
  arc A3814 (-19.1, 16.76) -> (-19.1, 16.66) centre (-19.1, 16.71) ccw
  arc A3815 (-18.9, 16.66) -> (-18.9, 16.76) centre (-18.9, 16.71) ccw
  line L1740 (-21.7, -26.6) -> (-21.7, -26.8)
  arc A3816 (-21.75, -26.8) -> (-21.65, -26.8) centre (-21.7, -26.8) ccw
  arc A3817 (-21.65, -26.6) -> (-21.75, -26.6) centre (-21.7, -26.6) ccw
  line L1741 (-21.7, -26.8) -> (-16.5, -26.8)
  arc A3818 (-16.5, -26.85) -> (-16.5, -26.75) centre (-16.5, -26.8) ccw
  arc A3819 (-21.7, -26.75) -> (-21.7, -26.85) centre (-21.7, -26.8) ccw
  line L1742 (-16.5, -26.8) -> (-16.5, -26.6)
  arc A3820 (-16.45, -26.6) -> (-16.55, -26.6) centre (-16.5, -26.6) ccw
  arc A3821 (-16.55, -26.8) -> (-16.45, -26.8) centre (-16.5, -26.8) ccw
  line L1743 (-16.5, -19.8) -> (-16.5, -19.6)
  arc A3822 (-16.45, -19.6) -> (-16.55, -19.6) centre (-16.5, -19.6) ccw
  arc A3823 (-16.55, -19.8) -> (-16.45, -19.8) centre (-16.5, -19.8) ccw
  line L1744 (-16.5, -19.6) -> (-21.7, -19.6)
  arc A3824 (-21.7, -19.55) -> (-21.7, -19.65) centre (-21.7, -19.6) ccw
  arc A3825 (-16.5, -19.65) -> (-16.5, -19.55) centre (-16.5, -19.6) ccw
  line L1745 (-21.7, -19.6) -> (-21.7, -19.8)
  arc A3826 (-21.75, -19.8) -> (-21.65, -19.8) centre (-21.7, -19.8) ccw
  arc A3827 (-21.65, -19.6) -> (-21.75, -19.6) centre (-21.7, -19.6) ccw
  line L1746 (-11.792, -118.758) -> (-11.792, -118.958)
  arc A3828 (-11.842, -118.958) -> (-11.742, -118.958) centre (-11.792, -118.958) ccw
  arc A3829 (-11.742, -118.758) -> (-11.842, -118.758) centre (-11.792, -118.758) ccw
  line L1747 (-11.792, -118.958) -> (-6.592, -118.958)
  arc A3830 (-6.592, -119.008) -> (-6.592, -118.908) centre (-6.592, -118.958) ccw
  arc A3831 (-11.792, -118.908) -> (-11.792, -119.008) centre (-11.792, -118.958) ccw
  line L1748 (-6.592, -118.958) -> (-6.592, -118.758)
  arc A3832 (-6.542, -118.758) -> (-6.642, -118.758) centre (-6.592, -118.758) ccw
  arc A3833 (-6.642, -118.958) -> (-6.542, -118.958) centre (-6.592, -118.958) ccw
  line L1749 (-6.592, -111.958) -> (-6.592, -111.758)
  arc A3834 (-6.542, -111.758) -> (-6.642, -111.758) centre (-6.592, -111.758) ccw
  arc A3835 (-6.642, -111.958) -> (-6.542, -111.958) centre (-6.592, -111.958) ccw
  line L1750 (-6.592, -111.758) -> (-11.792, -111.758)
  arc A3836 (-11.792, -111.708) -> (-11.792, -111.808) centre (-11.792, -111.758) ccw
  arc A3837 (-6.592, -111.808) -> (-6.592, -111.708) centre (-6.592, -111.758) ccw
  line L1751 (-11.792, -111.758) -> (-11.792, -111.958)
  arc A3838 (-11.842, -111.958) -> (-11.742, -111.958) centre (-11.792, -111.958) ccw
  arc A3839 (-11.742, -111.758) -> (-11.842, -111.758) centre (-11.792, -111.758) ccw
  line L1752 (-16.5, -67.942) -> (-16.5, -67.742)
  arc A3840 (-16.45, -67.742) -> (-16.55, -67.742) centre (-16.5, -67.742) ccw
  arc A3841 (-16.55, -67.942) -> (-16.45, -67.942) centre (-16.5, -67.942) ccw
  line L1753 (-16.5, -67.742) -> (-21.7, -67.742)
  arc A3842 (-21.7, -67.692) -> (-21.7, -67.792) centre (-21.7, -67.742) ccw
  arc A3843 (-16.5, -67.792) -> (-16.5, -67.692) centre (-16.5, -67.742) ccw
  line L1754 (-21.7, -67.742) -> (-21.7, -67.942)
  arc A3844 (-21.75, -67.942) -> (-21.65, -67.942) centre (-21.7, -67.942) ccw
  arc A3845 (-21.65, -67.742) -> (-21.75, -67.742) centre (-21.7, -67.742) ccw
  line L1755 (-21.7, -74.742) -> (-21.7, -74.942)
  arc A3846 (-21.75, -74.942) -> (-21.65, -74.942) centre (-21.7, -74.942) ccw
  arc A3847 (-21.65, -74.742) -> (-21.75, -74.742) centre (-21.7, -74.742) ccw
  line L1756 (-21.7, -74.942) -> (-16.5, -74.942)
  arc A3848 (-16.5, -74.992) -> (-16.5, -74.892) centre (-16.5, -74.942) ccw
  arc A3849 (-21.7, -74.892) -> (-21.7, -74.992) centre (-21.7, -74.942) ccw
  line L1757 (-16.5, -74.942) -> (-16.5, -74.742)
  arc A3850 (-16.45, -74.742) -> (-16.55, -74.742) centre (-16.5, -74.742) ccw
  arc A3851 (-16.55, -74.942) -> (-16.45, -74.942) centre (-16.5, -74.942) ccw
  line L1758 (-25.692, 17.3) -> (-25.692, 17.1)
  arc A3852 (-25.742, 17.1) -> (-25.642, 17.1) centre (-25.692, 17.1) ccw
  arc A3853 (-25.642, 17.3) -> (-25.742, 17.3) centre (-25.692, 17.3) ccw
  line L1759 (-25.692, 17.1) -> (-20.492, 17.1)
  arc A3854 (-20.492, 17.05) -> (-20.492, 17.15) centre (-20.492, 17.1) ccw
  arc A3855 (-25.692, 17.15) -> (-25.692, 17.05) centre (-25.692, 17.1) ccw
  line L1760 (-20.492, 17.1) -> (-20.492, 17.3)
  arc A3856 (-20.442, 17.3) -> (-20.542, 17.3) centre (-20.492, 17.3) ccw
  arc A3857 (-20.542, 17.1) -> (-20.442, 17.1) centre (-20.492, 17.1) ccw
  line L1761 (-20.492, 24.1) -> (-20.492, 24.3)
  arc A3858 (-20.442, 24.3) -> (-20.542, 24.3) centre (-20.492, 24.3) ccw
  arc A3859 (-20.542, 24.1) -> (-20.442, 24.1) centre (-20.492, 24.1) ccw
  line L1762 (-20.492, 24.3) -> (-25.692, 24.3)
  arc A3860 (-25.692, 24.35) -> (-25.692, 24.25) centre (-25.692, 24.3) ccw
  arc A3861 (-20.492, 24.25) -> (-20.492, 24.35) centre (-20.492, 24.3) ccw
  line L1763 (-25.692, 24.3) -> (-25.692, 24.1)
  arc A3862 (-25.742, 24.1) -> (-25.642, 24.1) centre (-25.692, 24.1) ccw
  arc A3863 (-25.642, 24.3) -> (-25.742, 24.3) centre (-25.692, 24.3) ccw
  line L1764 (1.208, -115.683) -> (1.408, -115.683)
  arc A3864 (1.408, -115.733) -> (1.408, -115.633) centre (1.408, -115.683) ccw
  arc A3865 (1.208, -115.633) -> (1.208, -115.733) centre (1.208, -115.683) ccw
  line L1765 (1.408, -115.683) -> (1.408, -110.483)
  arc A3866 (1.458, -110.483) -> (1.358, -110.483) centre (1.408, -110.483) ccw
  arc A3867 (1.358, -115.683) -> (1.458, -115.683) centre (1.408, -115.683) ccw
  line L1766 (1.408, -110.483) -> (1.208, -110.483)
  arc A3868 (1.208, -110.433) -> (1.208, -110.533) centre (1.208, -110.483) ccw
  arc A3869 (1.408, -110.533) -> (1.408, -110.433) centre (1.408, -110.483) ccw
  line L1767 (-5.592, -110.483) -> (-5.792, -110.483)
  arc A3870 (-5.792, -110.433) -> (-5.792, -110.533) centre (-5.792, -110.483) ccw
  arc A3871 (-5.592, -110.533) -> (-5.592, -110.433) centre (-5.592, -110.483) ccw
  line L1768 (-5.792, -110.483) -> (-5.792, -115.683)
  arc A3872 (-5.842, -115.683) -> (-5.742, -115.683) centre (-5.792, -115.683) ccw
  arc A3873 (-5.742, -110.483) -> (-5.842, -110.483) centre (-5.792, -110.483) ccw
  line L1769 (-5.792, -115.683) -> (-5.592, -115.683)
  arc A3874 (-5.592, -115.733) -> (-5.592, -115.633) centre (-5.592, -115.683) ccw
  arc A3875 (-5.792, -115.633) -> (-5.792, -115.733) centre (-5.792, -115.683) ccw
  line L1770 (-5.592, -53.66) -> (-5.792, -53.66)
  arc A3876 (-5.792, -53.61) -> (-5.792, -53.71) centre (-5.792, -53.66) ccw
  arc A3877 (-5.592, -53.71) -> (-5.592, -53.61) centre (-5.592, -53.66) ccw
  line L1771 (-5.792, -53.66) -> (-5.792, -58.86)
  arc A3878 (-5.842, -58.86) -> (-5.742, -58.86) centre (-5.792, -58.86) ccw
  arc A3879 (-5.742, -53.66) -> (-5.842, -53.66) centre (-5.792, -53.66) ccw
  line L1772 (-5.792, -58.86) -> (-5.592, -58.86)
  arc A3880 (-5.592, -58.91) -> (-5.592, -58.81) centre (-5.592, -58.86) ccw
  arc A3881 (-5.792, -58.81) -> (-5.792, -58.91) centre (-5.792, -58.86) ccw
  line L1773 (1.208, -58.86) -> (1.408, -58.86)
  arc A3882 (1.408, -58.91) -> (1.408, -58.81) centre (1.408, -58.86) ccw
  arc A3883 (1.208, -58.81) -> (1.208, -58.91) centre (1.208, -58.86) ccw
  line L1774 (1.408, -58.86) -> (1.408, -53.66)
  arc A3884 (1.458, -53.66) -> (1.358, -53.66) centre (1.408, -53.66) ccw
  arc A3885 (1.358, -58.86) -> (1.458, -58.86) centre (1.408, -58.86) ccw
  line L1775 (1.408, -53.66) -> (1.208, -53.66)
  arc A3886 (1.208, -53.61) -> (1.208, -53.71) centre (1.208, -53.66) ccw
  arc A3887 (1.408, -53.71) -> (1.408, -53.61) centre (1.408, -53.66) ccw
  line L1776 (1.208, 15.883) -> (1.408, 15.883)
  arc A3888 (1.408, 15.833) -> (1.408, 15.933) centre (1.408, 15.883) ccw
  arc A3889 (1.208, 15.933) -> (1.208, 15.833) centre (1.208, 15.883) ccw
  line L1777 (1.408, 15.883) -> (1.408, 21.083)
  arc A3890 (1.458, 21.083) -> (1.358, 21.083) centre (1.408, 21.083) ccw
  arc A3891 (1.358, 15.883) -> (1.458, 15.883) centre (1.408, 15.883) ccw
  line L1778 (1.408, 21.083) -> (1.208, 21.083)
  arc A3892 (1.208, 21.133) -> (1.208, 21.033) centre (1.208, 21.083) ccw
  arc A3893 (1.408, 21.033) -> (1.408, 21.133) centre (1.408, 21.083) ccw
  line L1779 (-5.592, 21.083) -> (-5.792, 21.083)
  arc A3894 (-5.792, 21.133) -> (-5.792, 21.033) centre (-5.792, 21.083) ccw
  arc A3895 (-5.592, 21.033) -> (-5.592, 21.133) centre (-5.592, 21.083) ccw
  line L1780 (-5.792, 21.083) -> (-5.792, 15.883)
  arc A3896 (-5.842, 15.883) -> (-5.742, 15.883) centre (-5.792, 15.883) ccw
  arc A3897 (-5.742, 21.083) -> (-5.842, 21.083) centre (-5.792, 21.083) ccw
  line L1781 (-5.792, 15.883) -> (-5.592, 15.883)
  arc A3898 (-5.592, 15.833) -> (-5.592, 15.933) centre (-5.592, 15.883) ccw
  arc A3899 (-5.792, 15.933) -> (-5.792, 15.833) centre (-5.792, 15.883) ccw
  line L1782 (-16.125, -38.375) -> (-13.675, -38.375)
  arc A3900 (-13.675, -38.4067) -> (-13.675, -38.3432) centre (-13.675, -38.375) ccw
  arc A3901 (-16.125, -38.3432) -> (-16.125, -38.4067) centre (-16.125, -38.375) ccw
  line L1783 (-13.675, -39.825) -> (-16.125, -39.825)
  arc A3902 (-16.125, -39.7932) -> (-16.125, -39.8567) centre (-16.125, -39.825) ccw
  arc A3903 (-13.675, -39.8567) -> (-13.675, -39.7932) centre (-13.675, -39.825) ccw
  line L1784 (-16.125, -39.825) -> (-16.125, -38.375)
  arc A3904 (-16.0933, -38.375) -> (-16.1568, -38.375) centre (-16.1251, -38.375) ccw
  arc A3905 (-16.1568, -39.825) -> (-16.0933, -39.825) centre (-16.1251, -39.825) ccw
  line L1785 (-13.675, -38.375) -> (-13.675, -39.825)